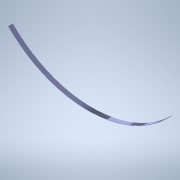
# Autodesk Inventor part: Chapa_Calço_Curvada
Saved by Autodesk Inventor 2022 (Build 260153000, 153)
## iProperties
Created: 2016-02-19
Part Number: Chapa_Calço_Curvada
Material: Genérico
Document SubType Name: Modeling
Designer: al131100X
Density: 1 g/cm^3
Appearance: Padrão
Author: al131100X
Autodesk Inventor part; units mm, degrees
ref_plane "YZ Plane" through (0, 0, 0) normal (1, 0, 0) x (0, 1, 0)
ref_plane "XZ Plane" through (0, 0, 0) normal (0, 1, 0) x (-1, 0, 0)
ref_plane "XY Plane" through (0, 0, 0) normal (0, 0, 1) x (1, 0, 0)
sketch "Sketch1" plane through (0, 0, 0) normal (0, 1, 0) x (-1, 0, 0)
  arc A0 (2077.4812, 261.4133) -> (3881.9735, 263.7927) centre (2978.5428, 1160.9837) ccw
  arc A1 (2079.7282, 263.6565) -> (3879.7266, 266.0359) centre (2978.5428, 1160.9837) ccw
  line L0 (3881.9735, 263.7927) -> (3879.7266, 266.0359)
  line L1 (2077.4812, 261.4133) -> (2079.7282, 263.6565)
  point P0 (0, 0)
  dimension "d0" = 2546.4791
  dimension "d9" = 3.175
  dimension "d16" = 1800
  constraints: 4 end point, 4 point on circle, 2 centre point, 1 other
  measures "d0" diameter of A0
  measures "d9" radial gap between concentric circles of A0 A1
  measures "d16" distance of L0.end L1.end
extrude "Extrusion1" add sketch "Sketch1" along normal blind 50.8
body "Solid1"
